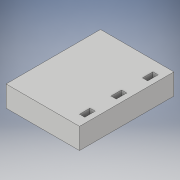
# Autodesk Inventor part: LEDBottom
Saved by Autodesk Inventor 2019 (Build 230136000, 136)
## iProperties
Created: 2018-12-07
Part Number: LEDBottom
Material: Generic
Document SubType Name: Modeling
Designer: Administrator
Density: 1 g/cm^3
Appearance: Default
Author: Administrator
Autodesk Inventor part; units mm, degrees
ref_plane "YZ Plane" through (0, 0, 0) normal (1, 0, 0) x (0, 1, 0)
ref_plane "XZ Plane" through (0, 0, 0) normal (0, 1, 0) x (-1, 0, 0)
ref_plane "XY Plane" through (0, 0, 0) normal (0, 0, 1) x (1, 0, 0)
sketch "Sketch1" plane through (0, 0, 0) normal (0, 1, 0) x (-1, 0, 0)
  line L0 (0, 0) -> (88.9, 0)
  line L1 (88.9, 0) -> (88.9, -114.3)
  line L2 (88.9, -114.3) -> (0, -114.3)
  line L3 (0, -114.3) -> (0, 0)
  line L4 (6.35, -12.7) -> (12.7, -12.7)
  line L5 (12.7, -12.7) -> (12.7, -25.4)
  line L6 (12.7, -25.4) -> (6.35, -25.4)
  line L7 (6.35, -25.4) -> (6.35, -12.7)
  line L8 (12.7, -88.9) -> (6.35, -88.9)
  line L9 (6.35, -88.9) -> (6.35, -101.6)
  line L10 (6.35, -101.6) -> (12.7, -101.6)
  line L11 (12.7, -101.6) -> (12.7, -88.9)
  line L12 (12.7, -50.8) -> (6.35, -50.8)
  line L13 (6.35, -50.8) -> (6.35, -63.5)
  line L14 (6.35, -63.5) -> (12.7, -63.5)
  line L15 (12.7, -63.5) -> (12.7, -50.8)
  dimension "d0" = 88.9
  dimension "d1" = 114.3
  dimension "d2" = 6.35
  dimension "d3" = 12.7
  dimension "d4" = 6.35
  dimension "d5" = 12.7
  dimension "d6" = 12.7
  dimension "d7" = 12.7
  dimension "d8" = 12.7
  dimension "d9" = 63.5
  dimension "d10" = 25.4
  dimension "d11" = 25.4
  constraints: 32 end point, 8 parallel, 4 horizontal, 4 perpendicular
  measures "d0" distance of L1.end L2.end
  measures "d1" distance of L0.end L1.end
  measures "d2" distance of L5.end L6.end
  measures "d3" distance of L4.end L5.end
  measures "d4" distance between parallel lines of L3 L7
  measures "d5" distance between parallel lines of L0 L4
  measures "d6" distance of L9.end L8.end
  measures "d7" distance between parallel lines of L2 L10
  measures "d8" distance of L14.end L12.start
  measures "d9" distance between parallel lines of L8 L6
  measures "d10" distance between parallel lines of L12 L6
  measures "d11" distance between parallel lines of L8 L14
extrude "Extrusion1" add sketch "Sketch1" along normal blind 25.4
body "Solid1"
